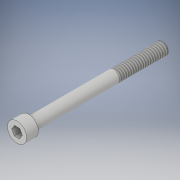
# Autodesk Inventor part: 10 l 20 2 1 l 2 bolt
Saved by Autodesk Inventor 2018 (Build 220112000, 112)
## iProperties
Created: 2019-03-20
Part Number: 10 l 20 2 1 l 2 bolt
Material: Generic
Document SubType Name: Modeling
Designer: S-4008082
Density: 1 g/cm^3
Appearance: Default
Author: S-4008082
Autodesk Inventor part; units mm, degrees
ref_plane "YZ Plane" through (0, 0, 0) normal (1, 0, 0) x (0, 1, 0)
ref_plane "XZ Plane" through (0, 0, 0) normal (0, 1, 0) x (-1, 0, 0)
ref_plane "XY Plane" through (0, 0, 0) normal (0, 0, 1) x (1, 0, 0)
sketch "Sketch1" plane through (0, 0, 0) normal (0, 0, 1) x (1, 0, 0)
  circle A0 centre (0, 0) radius 2.5797
  dimension "d0" = 5.1594
  constraints: 1 centre point, 1 coincident
  measures "d0" diameter of A0
extrude "Extrusion1" add sketch "Sketch1" along normal blind 58.42
sketch "Sketch2" plane through (0, 0, 58.42) normal (0, 0, 1) x (1, 0, 0)
  circle A0 centre (0, 0) radius 4.1967
  constraints: 1 centre point, 1 coincident
extrude "Extrusion2" add sketch "Sketch2" along normal blind 5.08
sketch "Sketch3" plane through (0, 0, 63.5) normal (0, 0, 1) x (1, 0, 0)
  line L0 (1.1457, 1.9844) -> (2.2914, 0)
  line L1 (2.2914, 0) -> (1.1457, -1.9844)
  line L2 (1.1457, -1.9844) -> (-1.1457, -1.9844)
  line L3 (-1.1457, -1.9844) -> (-2.2914, 0)
  line L4 (-2.2914, 0) -> (-1.1457, 1.9844)
  line L5 (-1.1457, 1.9844) -> (1.1457, 1.9844)
  point P0 (0, 0)
  point P1 (0, 0)
  point P2 (0, 1.9844)
  dimension "d5" = 3.9688
  constraints: 12 end point, 1 coincident, 1 midpoint, 13 other
  measures "d5" distance between parallel lines of L4 L1
extrude "Extrusion3" cut sketch "Sketch3" against normal blind 4.445
thread "Thread1" size "12-24 UNC" class "2A" standard "ANSI Unified Screw Threads" length 21.59
fillet "Fillet1" radius 0.254 1 edges at (-2.5797, 0, 0)
body "Solid1"
